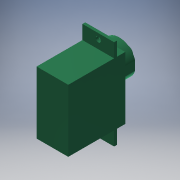
# Autodesk Inventor part: HS55
Saved by Autodesk Inventor 2016 (Build 200138000, 138)
## iProperties
Created: 2015-08-04
Part Number: HS55
Material: Generic
Document SubType Name: Modeling
Designer: lk8187
Density: 1 g/cm^3
Appearance: Smooth - Dark Sea Green
Author: lk8187
Autodesk Inventor part; units mm, degrees
ref_plane "YZ Plane" through (0, 0, 0) normal (1, 0, 0) x (0, 1, 0)
ref_plane "XZ Plane" through (0, 0, 0) normal (0, 1, 0) x (-1, 0, 0)
ref_plane "XY Plane" through (0, 0, 0) normal (0, 0, 1) x (1, 0, 0)
sketch "Sketch1" plane through (0, 0, 0) normal (0, 1, 0) x (-1, 0, 0)
  line L0 (-5.705, 6) -> (5.705, 6)
  line L1 (5.705, 6) -> (5.705, -16.48)
  line L2 (5.705, -16.48) -> (-5.705, -16.48)
  line L3 (-5.705, -16.48) -> (-5.705, 6)
  line L4 (-5.705, 11.035) -> (5.705, 11.035)
  line L5 (5.705, 11.035) -> (5.705, -21.515)
  line L6 (5.705, -21.515) -> (-5.705, -21.515)
  line L7 (-5.705, -21.515) -> (-5.705, 11.035)
  circle A0 centre (0, 0) radius 2
  line L8 (0, 9.0475) -> (0, 11.035) construction
  line L9 (0, -19.5275) -> (0, -21.515) construction
  line L10 (-5.705, 6) -> (-5.705, 11.035) construction
  line L11 (-5.705, -16.48) -> (-5.705, -21.515) construction
  arc A1 (5.705, 1.6543) -> (-5.705, 1.6543) centre (0, 0) ccw
  arc A2 (-5.705, -1.6543) -> (5.705, -1.6543) centre (0, 0) ccw
  line L12 (5.705, 11.035) -> (-5.705, 11.035)
  line L13 (-5.705, 11.035) -> (-5.705, 6)
  line L14 (-5.705, 6) -> (5.705, 6)
  line L15 (5.705, 6) -> (5.705, 11.035)
  line L16 (5.705, -16.48) -> (-5.705, -16.48)
  line L17 (-5.705, -16.48) -> (-5.705, -21.515)
  line L18 (-5.705, -21.515) -> (5.705, -21.515)
  line L19 (5.705, -21.515) -> (5.705, -16.48)
  point P0 (0, 6)
  dimension "d0" = 11.41
  dimension "d8" = 32.55
  dimension "d10" = 4
  dimension "d28" = 22.48
  dimension "d29" = 6
  dimension "d30" = 28.575
  dimension "d31" = 5.94
  constraints: 40 end point, 8 parallel, 8 perpendicular, 6 point on line, 4 horizontal, 4 midpoint, 4 point on circle, 4 vertical alignment, 3 centre point, 3 collinear, 2 coincident, 1 concentric
  measures "d0" distance of L4.start L4.end
  measures "d8" distance between parallel lines of L6 L4
  measures "d10" diameter of A0
  measures "d28" distance between parallel lines of L0 L2
  measures "d29" distance from line of point (0, 0) L0
  measures "d30" distance of L9.start L8.start
  measures "d31" radius of A2
extrude "Extrusion1" add sketch "Sketch1" along normal blind 4 and the other way blind 16.52 contours L0 L1 A1 L3 | A1 L1 A2 L3 | A2 L1 L2 L3 | A0
extrude "Extrusion5" add sketch "Sketch1" along normal blind 1 contours L7 L4 L5 L0 | L2 L5 L6 L7
extrude "Extrusion3" add sketch "Sketch1" along normal blind 7.56 contours A1 L1 A2 L3
extrude "Extrusion4" add sketch "Sketch1" along normal blind 10.56 contours A0
hole "Hole1" at (0, 0, 9.0475) at (0, 0, -19.5275) direction (0, 1, 0) diameter 1.8 end through all
body "Solid1"
